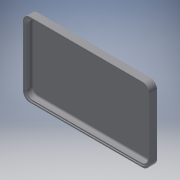
# Autodesk Inventor part: Hub Enclosure
Saved by Autodesk Inventor 2018 (Build 220112000, 112)
## iProperties
Created: 2018-03-22
Part Number: Hub Enclosure
Material: Generic
Document SubType Name: Modeling
Designer: brutu
Density: 1 g/cm^3
Appearance: Default
Author: brutu
Autodesk Inventor part; units mm, degrees
ref_plane "YZ Plane" through (0, 0, 0) normal (1, 0, 0) x (0, 1, 0)
ref_plane "XZ Plane" through (0, 0, 0) normal (0, 1, 0) x (-1, 0, 0)
ref_plane "XY Plane" through (0, 0, 0) normal (0, 0, 1) x (1, 0, 0)
sketch "Sketch1" plane through (0, 0, 0) normal (0, 0, 1) x (1, 0, 0)
  line L0 (77.5, 43.5) -> (77.5, -43.5) projected
  line L1 (77.5, -43.5) -> (-77.5, -43.5) projected
  line L2 (-77.5, -43.5) -> (-77.5, 43.5) projected
  line L3 (-77.5, 43.5) -> (77.5, 43.5) projected
  line L4 (85.48, 55.38) -> (-85.48, 55.38) projected
  arc A0 (-85.48, 55.38) -> (-96.48, 44.38) centre (-85.48, 44.38) ccw projected
  line L5 (-96.48, 44.38) -> (-96.48, -44.38) projected
  arc A1 (-96.48, -44.38) -> (-85.48, -55.38) centre (-85.48, -44.38) ccw projected
  line L6 (-85.48, -55.38) -> (85.48, -55.38) projected
  arc A2 (85.48, -55.38) -> (96.48, -44.38) centre (85.48, -44.38) ccw projected
  line L7 (96.48, -44.38) -> (96.48, 44.38) projected
  arc A3 (96.48, 44.38) -> (85.48, 55.38) centre (85.48, 44.38) ccw projected
  line L8 (-88.48, 58.38) -> (88.48, 58.38)
  line L9 (99.48, 47.38) -> (99.48, -47.38)
  line L10 (88.48, -58.38) -> (-88.48, -58.38)
  line L11 (-99.48, -47.38) -> (-99.48, 47.38)
  arc A4 (-88.48, 58.38) -> (-99.48, 47.38) centre (-88.48, 47.38) ccw
  arc A5 (99.48, 47.38) -> (88.48, 58.38) centre (88.48, 47.38) ccw
  arc A6 (88.48, -58.38) -> (99.48, -47.38) centre (88.48, -47.38) ccw
  arc A7 (-99.48, -47.38) -> (-88.48, -58.38) centre (-88.48, -47.38) ccw
  point P0 (0, 0)
  dimension "d0" = 3
  dimension "d1" = 3
  dimension "d2" = 3
  dimension "d3" = 3
  dimension "d4" = 11
  dimension "d5" = 11
  constraints: 8 end point, 8 point on circle, 8 tangent, 4 centre point, 3 equal radius, 2 parallel, 1 horizontal, 1 perpendicular
  measures "d0" distance between parallel lines of L5 L11
  measures "d1" distance between parallel lines of L4 L8
  measures "d2" distance between parallel lines of L9 L7
  measures "d3" distance between parallel lines of L10 L6
  measures "d4" radius of A4
  measures "d5" radius of A0
extrude "Extrusion1" add sketch "Sketch1" against normal blind 12 contours L0 L1 L2 L3 | A3 L7 A2 L6 A1 L5 A0 L4 | L8 A5 L9 A6 L10 A7 L11 A4
sketch "Sketch2" plane through (0, 0, 0) normal (0, 0, 1) x (1, 0, 0)
  line L0 (-88.48, 58.38) -> (88.48, 58.38) projected
  arc A0 (-88.48, 58.38) -> (-99.48, 47.38) centre (-88.48, 47.38) ccw projected
  line L1 (-99.48, -47.38) -> (-99.48, 47.38) projected
  arc A1 (-99.48, -47.38) -> (-88.48, -58.38) centre (-88.48, -47.38) ccw projected
  line L2 (88.48, -58.38) -> (-88.48, -58.38) projected
  arc A2 (88.48, -58.38) -> (99.48, -47.38) centre (88.48, -47.38) ccw projected
  line L3 (99.48, 47.38) -> (99.48, -47.38) projected
  arc A3 (99.48, 47.38) -> (88.48, 58.38) centre (88.48, 47.38) ccw projected
  line L4 (77.5, 43.5) -> (77.5, -43.5) projected
  line L5 (77.5, -43.5) -> (-77.5, -43.5) projected
  line L6 (-77.5, -43.5) -> (-77.5, 43.5) projected
  line L7 (-77.5, 43.5) -> (77.5, 43.5) projected
  line L8 (85.48, 55.38) -> (-85.48, 55.38) projected
  arc A4 (-85.48, 55.38) -> (-96.48, 44.38) centre (-85.48, 44.38) ccw projected
  line L9 (-96.48, 44.38) -> (-96.48, -44.38) projected
  arc A5 (-96.48, -44.38) -> (-85.48, -55.38) centre (-85.48, -44.38) ccw projected
  line L10 (-85.48, -55.38) -> (85.48, -55.38) projected
  arc A6 (85.48, -55.38) -> (96.48, -44.38) centre (85.48, -44.38) ccw projected
  line L11 (96.48, -44.38) -> (96.48, 44.38) projected
  arc A7 (96.48, 44.38) -> (85.48, 55.38) centre (85.48, 44.38) ccw projected
  arc A8 (-85.48, 56.38) -> (-97.48, 44.38) centre (-85.48, 44.38) ccw
  line L12 (-85.48, 56.38) -> (85.48, 56.38)
  arc A9 (97.48, 44.38) -> (85.48, 56.38) centre (85.48, 44.38) ccw
  line L13 (97.48, 44.38) -> (97.48, -44.38)
  arc A10 (85.48, -56.38) -> (97.48, -44.38) centre (85.48, -44.38) ccw
  line L14 (85.48, -56.38) -> (-85.48, -56.38)
  arc A11 (-97.48, -44.38) -> (-85.48, -56.38) centre (-85.48, -44.38) ccw
  line L15 (-97.48, -44.38) -> (-97.48, 44.38)
  point P0 (0, 0)
  dimension "d8" = 1
  constraints: 8 end point, 8 point on circle, 4 centre point, 7 other
  measures "d8" radial gap between concentric circles of A4 A8
extrude "Extrusion2" cut sketch "Sketch2" against normal blind 1.5 contours L4 L5 L6 L7 | A7 L11 A6 L10 A5 L9 A4 L8 | L12 A9 L13 A10 L14 A11 L15 A8
sketch "Sketch3" plane through (0, 0, -1.5) normal (0, 0, 1) x (1, 0, 0)
  arc A0 (-85.48, 56.38) -> (-97.48, 44.38) centre (-85.48, 44.38) ccw projected
  line L0 (-97.48, -44.38) -> (-97.48, 44.38) projected
  arc A1 (-97.48, -44.38) -> (-85.48, -56.38) centre (-85.48, -44.38) ccw projected
  line L1 (85.48, -56.38) -> (-85.48, -56.38) projected
  arc A2 (85.48, -56.38) -> (97.48, -44.38) centre (85.48, -44.38) ccw projected
  line L2 (97.48, 44.38) -> (97.48, -44.38) projected
  arc A3 (97.48, 44.38) -> (85.48, 56.38) centre (85.48, 44.38) ccw projected
  line L3 (-85.48, 56.38) -> (85.48, 56.38) projected
  arc A4 (-85.48, 54.38) -> (-95.48, 44.38) centre (-85.48, 44.38) ccw
  line L4 (-85.48, 54.38) -> (85.48, 54.38)
  arc A5 (95.48, 44.38) -> (85.48, 54.38) centre (85.48, 44.38) ccw
  line L5 (95.48, 44.38) -> (95.48, -44.38)
  arc A6 (85.48, -54.38) -> (95.48, -44.38) centre (85.48, -44.38) ccw
  line L6 (85.48, -54.38) -> (-85.48, -54.38)
  arc A7 (-95.48, -44.38) -> (-85.48, -54.38) centre (-85.48, -44.38) ccw
  line L7 (-95.48, -44.38) -> (-95.48, 44.38)
  point P0 (0, 0)
  dimension "d11" = 2
  constraints: 8 end point, 8 point on circle, 4 centre point, 7 other
  measures "d11" radial gap between concentric circles of A0 A4
extrude "Extrusion3" cut sketch "Sketch3" against normal blind 8 contours L4 A5 L5 A6 L6 A7 L7 A4
fillet "Fillet1" radius 3.175 8 edges at (92.5511, 51.4511, -9.5) (95.48, 0, -9.5) (92.5511, -51.4511, -9.5) (0, -54.38, -9.5) (-92.5511, -51.4511, -9.5) (-95.48, 0, -9.5) (-92.5511, 51.4511, -9.5) (0, 54.38, -9.5)
sketch "Sketch4" plane through (0, 0, -12) normal (0, 0, -1) x (-1, 0, 0)
  line L0 (-35.15, 31.45) -> (43.7742, 31.45) projected
  arc A0 (46.7742, 28.45) -> (43.7742, 31.45) centre (43.7742, 28.45) ccw projected
  line L1 (46.7742, 28.45) -> (46.7742, -21.55) projected
  arc A1 (43.7742, -24.55) -> (46.7742, -21.55) centre (43.7742, -21.55) ccw projected
  line L2 (43.7742, -24.55) -> (-35.15, -24.55) projected
  arc A2 (-38.15, -21.55) -> (-35.15, -24.55) centre (-35.15, -21.55) ccw projected
  line L3 (-38.15, -21.55) -> (-38.15, 28.45) projected
  arc A3 (-35.15, 31.45) -> (-38.15, 28.45) centre (-35.15, 28.45) ccw projected
  line L4 (-48.26, 38.1) -> (48.26, 38.1)
  line L5 (50.8, 35.56) -> (50.8, -35.56)
  line L6 (48.26, -38.1) -> (-48.26, -38.1)
  line L7 (-50.8, -35.56) -> (-50.8, 35.56)
  arc A4 (-48.26, 38.1) -> (-50.8, 35.56) centre (-48.26, 35.56) ccw
  arc A5 (50.8, 35.56) -> (48.26, 38.1) centre (48.26, 35.56) ccw
  arc A6 (48.26, -38.1) -> (50.8, -35.56) centre (48.26, -35.56) ccw
  arc A7 (-50.8, -35.56) -> (-48.26, -38.1) centre (-48.26, -35.56) ccw
  point P0 (0, 0)
  point P1 (-50.8, 38.1)
  point P2 (50.8, 38.1)
  point P3 (-50.8, -38.1)
  dimension "d15" = 101.6
  dimension "d16" = 76.2
  dimension "d17" = 38.1
  dimension "d18" = 50.8
  dimension "d19" = 2.54
  constraints: 8 end point, 8 point on circle, 8 tangent, 6 point on line, 4 centre point, 3 equal radius, 2 parallel, 1 horizontal, 1 perpendicular
  measures "d15" distance of point (-50.8, 38.1) point (50.8, 38.1)
  measures "d16" distance of point (-50.8, -38.1) point (-50.8, 38.1)
  measures "d17" distance from line of point (0, 0) L4
  measures "d18" distance from line of L7 point (0, 0)
  measures "d19" radius of A4
equation "\"d1\" = d0"
equation "\"d2\" = d0"
equation "\"d3\" = d0"
equation "\"d4\" = d5"
equation "\"d17\" = 0.5 * d16"
equation "\"d18\" = 0.5 * d15"
body "Solid1"
